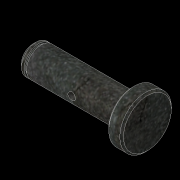
# Autodesk Inventor part: KON_Nietmaschine_Bolzen
Saved by Autodesk Inventor 2019 (Build 230136000, 136)
## iProperties
Created: 2021-11-08
Part Number: KON_Nietmaschine_Bolzen
Material: Stahl
Document SubType Name: Modeling
Designer: Jonas Nebl
Mass: 116.129 g
Surface Area: 52.2032 cm^2
Volume: 14.7935 cm^3
Density: 7.85 g/cm^3
Appearance: Platte
Author: Jonas Nebl
Autodesk Inventor part; units mm, degrees
ref_plane "YZ Plane" through (0, 0, 0) normal (1, 0, 0) x (0, 1, 0)
ref_plane "XZ Plane" through (0, 0, 0) normal (0, 1, 0) x (-1, 0, 0)
sketch "Skizze1" plane through (0, 0, 0) normal (0, 0, 1) x (1, 0, 0)
  line L0 (-31.2, 0) -> (-31.2, 8)
  line L1 (-31.2, 8) -> (-27.8, 8)
  line L2 (-27.8, 8) -> (-27.8, 7.15)
  line L3 (-27.8, 7.15) -> (-26.5, 7.15)
  line L4 (-26.5, 7.15) -> (-26.5, 8)
  line L5 (-26.5, 8) -> (23.2, 8)
  line L6 (23.2, 8) -> (23.2, 14)
  line L7 (23.2, 14) -> (31.2, 14)
  line L8 (31.2, 14) -> (31.2, 0)
  line L9 (-43.68, 0) -> (43.68, 0) projected
  line L10 (0, -2.8) -> (0, 16.8) projected
  line L11 (-31.2, 0) -> (31.2, 0)
  point P0 (0, 0)
  dimension "d0" = 49.7
  dimension "d1" = 8
  dimension "d2" = 6
  dimension "d3" = 1.3
  dimension "d4" = 0.85
  dimension "d5" = 3.4
  dimension "d6" = 8
  constraints: 20 end point, 4 point on line, 3 horizontal, 3 parallel, 3 vertical, 1 other
  measures "d0" distance between parallel lines of L6 L4
  measures "d1" distance of L6.end L7.end
  measures "d2" distance of L5.end L6.end
  measures "d3" distance between parallel lines of L4 L2
  measures "d4" distance of L3.end L4.end
  measures "d5" distance between parallel lines of L0 L2
  measures "d6" distance between parallel lines of L9 L5
revolve "Umdrehung1" add sketch "Skizze1" angle 360 about axis through (-10, 0, 0) along (1, 0, 0)
chamfer "Fase1" distance 2 angle 45 1 edges at (-31.2, -8, 0)
chamfer "Fase2" distance 1 angle 45 1 edges at (31.2, -14, 0)
chamfer "Fase3" distance 1 angle 45 1 edges at (23.2, -14, 0)
sketch "Skizze4" plane through (-31.2, 0, 0) normal (-1, 0, 0) x (0, 0, 1)
  point P0 (0, 0)
  point P1 (0, 0)
  constraints: 1 coincident
hole "Bohrung2" at (-31.2, 0, 0) direction (1, 0, 0) diameter 5 depth 35 tip angle 118
ref_plane "Arbeitsebene1" through (0, 0, 8) normal (0, 0, 1) x (1, 0, 0)
sketch "Skizze5" plane through (0, 0, 8) normal (0, 0, 1) x (1, 0, 0)
  line L0 (-2.4, 0) -> (0.4, 0) projected
  point P0 (0, 0)
  point P1 (-2, 0)
  dimension "d46" = 2
  constraints: 1 point on line
  measures "d46" distance of point (0, 0) point (-2, 0)
hole "Bohrung3" at (-2, 0, 8) direction (0, 0, -1) diameter 4 end through all
thread "Gewinde1" size "M5x0.8" class "6H" standard "ANSI Metric M Profile" length 15
